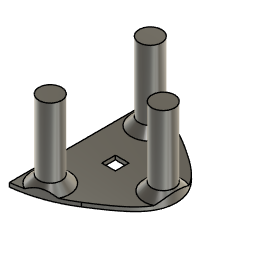
DirectionEncoderColumnSupport_PESTA (Autodesk Fusion 360 design; units mm, degrees)
Autodesk Fusion 360 part; units mm, degrees
note: some values were not read from the file. Set by a fixed rule: which sketch regions a step uses.
sketch "Sketch1" plane through (0, 0, 0) normal (0, 0, 1) x (1, 0, 0) in component "SuportePilarCentral"
  line L0 (39.35, 52.3) -> (-39.35, 52.3)
  line L1 (-39.35, 52.3) -> (-39.35, -52.3)
  line L2 (-39.35, -52.3) -> (39.35, -52.3)
  line L3 (39.35, -52.3) -> (39.35, 52.3)
  line L4 (39.35, 52.3) -> (-39.35, -52.3) construction
  line L5 (-39.35, 52.3) -> (39.35, -52.3) construction
  dimension "d1" = 78.7
  dimension "d2" = 104.6
  constraint horizontal L0
  constraint perpendicular L0 L1
  constraint parallel L0 L2
  constraint parallel L1 L3
  constraint coincident L4 origin
  constraint coincident L5 origin
  measures "d1" distance of L1.end L2.end
  measures "d2" distance of L0.end L1.end
extrude "Extrude1" add sketch "Sketch1" along normal blind 3 in component "SuportePilarCentral"
sketch "Sketch2" plane through (0, 0, 3) normal (0, 0, 1) x (-1, 0, 0) in component "SuportePilarCentral"
  line L0 (-39.35, 52.3) -> (-39.35, -52.3)
  line L1 (-39.35, -52.3) -> (39.35, -52.3)
  line L2 (39.35, -52.3) -> (39.35, 52.3)
  line L3 (39.35, 52.3) -> (-39.35, 52.3)
  circle A0 centre (23.55, -37.5) radius 8.5
  circle A1 centre (23.55, 37.5) radius 8.5
  line L4 (23.55, 37.5) -> (-23.65, 0)
  line L5 (-23.65, 0) -> (23.55, -37.5)
  circle A2 centre (-23.65, 0) radius 8.5
  dimension "d5" = 17
  dimension "d6" = 17
  dimension "d8" = 14.8
  dimension "d10" = 75
  dimension "d11" = 15.8
  dimension "d12" = 15.7
  dimension "d13" = 14.8
  dimension "d14" = 17
  constraint vertical A0.centre A1.centre
  constraint coincident A1.centre L4.start
  constraint coincident A0.centre L5.end
  constraint equal L4 L5
  constraint coincident L4.end L5.start
  measures "d5" diameter of A0
  measures "d6" diameter of A1
  measures "d8" distance of L3 A1.centre
  measures "d10" distance of A0.centre A1.centre
  measures "d11" distance of L2 A0.centre
  measures "d12" distance of L0 L4.end
  measures "d13" distance of L1 A0.centre
  measures "d14" diameter of A2
extrude "Extrude2" add sketch "Sketch2" along normal blind 58 contours A0 | A1 | L4 L5 A2 | L4 L5 A2 in component "SuportePilarCentral"
sketch "Sketch3" plane through (0, 0, 3) normal (0, 0, 1) x (-1, 0, 0) in component "SuportePilarCentral"
  circle A0 centre (23.55, 37.5) radius 8.5
  circle A1 centre (-23.65, 0) radius 8.5
  circle A2 centre (23.55, -37.5) radius 8.5
  line L0 (-39.35, 52.3) -> (-39.35, -52.3)
  line L1 (-39.35, -52.3) -> (39.35, -52.3)
  line L2 (39.35, -52.3) -> (39.35, 52.3)
  line L3 (39.35, 52.3) -> (-39.35, 52.3)
  spline S0 degree 5 poles (22.6923, -52.3) (20.9712, -51.282) (17.5667, -49.2595) (12.5727, -46.2662) (6.1404, -42.3567) (-1.5034, -37.5955) (-8.7027, -32.927) (-15.368, -28.2811) (-21.358, -23.5391) (-26.4613, -18.515) (-30.4038, -12.9641) (-32.9147, -6.7761) (-33.7822, 0) (-32.9147, 6.7761) (-30.4038, 12.9641) (-26.4613, 18.515) (-21.358, 23.5391) (-15.368, 28.2811) (-8.7027, 32.927) (-1.5034, 37.5955) (6.1404, 42.3567) (12.5727, 46.2662) (17.5667, 49.2595) (20.9712, 51.282) (22.6923, 52.3) knots 0 0 0 0 0 0 0.05 0.1 0.15 0.2 0.25 0.3 0.35 0.4 0.45 0.5 0.55 0.6 0.65 0.7 0.75 0.8 0.85 0.9 0.95 1 1 1 1 1 1
  line L4 (-33.35, -11.7865) -> (-33.35, 11.7865)
  point P0 (-19.35, -25)
  point P1 (-33.35, 0)
  point P2 (-19.35, 25)
  dimension "d17" = 25
  dimension "d18" = 25
  dimension "d19" = 6
  dimension "d20" = 20
  constraint coincident L1 S0.start
  constraint coincident L3 S0.end
  constraint vertical P0 P2
  constraint midpoint P1 L4
  constraint vertical L4
  constraint horizontal origin P1
  measures "d17" vertical distance of P0 P1
  measures "d18" vertical distance of P1 P2
  measures "d19" distance of L0 P1
  measures "d20" distance of L0 P0
extrude "Extrude3" cut sketch "Sketch3" against normal blind 3 contours L0 L1 L3 S0 in component "SuportePilarCentral"
fillet "Fillet1" radius 95 2 edges at (-22.6923, 52.3, 1.5) (-22.6923, -52.3, 1.5) in component "SuportePilarCentral"
sketch "Sketch4" plane through (0, 0, 3) normal (0, 0, 1) x (-1, 0, 0) in component "SuportePilarCentral"
  spline S0 degree 3 poles (-0.4688, 38.2043) (5.5357, 42.0059) (11.9479, 45.1218) (25.3467, 49.8648) (32.291, 51.4772) (39.35, 52.3) knots 0 0 0 0 2.132026 2.132026 4.264052 4.264052 4.264052 4.264052
  spline S1 degree 5 poles (-0.4688, 38.2043) (-0.6541, 38.087) (-2.3306, 37.0243) (-5.4453, 35.0269) (-9.8704, 32.1131) (-15.368, 28.2811) (-21.358, 23.5391) (-26.4613, 18.515) (-30.4038, 12.9641) (-32.9147, 6.7761) (-33.7822, 0) (-32.9147, -6.7761) (-30.4038, -12.9641) (-26.4613, -18.515) (-21.358, -23.5391) (-15.368, -28.2811) (-9.8704, -32.1131) (-5.4453, -35.0269) (-2.3306, -37.0243) (-0.6541, -38.087) (-0.4688, -38.2043) knots -0.856201 -0.856201 -0.856201 -0.856201 -0.856201 -0.856201 -0.85 -0.8 -0.75 -0.7 -0.65 -0.6 -0.55 -0.5 -0.45 -0.4 -0.35 -0.3 -0.25 -0.2 -0.15 -0.143799 -0.143799 -0.143799 -0.143799 -0.143799 -0.143799
  spline S2 degree 3 poles (39.35, -52.3) (37.5871, -52.0945) (34.0728, -51.5847) (28.8525, -50.5259) (23.6998, -49.1763) (18.6307, -47.5402) (13.6612, -45.6227) (8.8069, -43.4298) (4.0831, -40.9685) (1.0308, -39.1537) (-0.4688, -38.2043) knots 0 0 0 0 0.125 0.25 0.375 0.5 0.625 0.75 0.875 1 1 1 1
  line L0 (39.35, -52.3) -> (39.35, 52.3)
  circle A0 centre (23.55, -37.5) radius 8.5
  circle A1 centre (-23.65, 0) radius 8.5
  circle A2 centre (23.55, 37.5) radius 8.5
  line L1 (17.35, -5.1) -> (7.15, -5.1)
  line L2 (7.15, -5.1) -> (7.15, 5.1)
  line L3 (7.15, 5.1) -> (17.35, 5.1)
  line L4 (17.35, 5.1) -> (17.35, -5.1)
  point P0 (7.15, 0)
  dimension "d25" = 10.2
  dimension "d26" = 10.2
  dimension "d27" = 22
  constraint horizontal L1
  constraint vertical L2
  constraint horizontal L3
  constraint vertical L4
  constraint midpoint L2 P0
  constraint horizontal origin P0
  measures "d25" distance of L1.start L1.end
  measures "d26" distance of L1.start L3.end
  measures "d27" distance of L0 L4
extrude "Extrude4" cut sketch "Sketch4" against normal blind 3 contours L1 L2 L3 L4 in component "SuportePilarCentral"
chamfer "Chamfer1" distance 6 angle 45 3 edges at (-15.6252, 34.4263, 3) (-15.6252, -40.5737, 3) (31.5748, -3.0737, 3) in component "SuportePilarCentral"
component "SuportePilarCentral" placed x (1, 0, 0) y (0, 1, 0) z (0, 0, 1) at (0, 0, 0)
equation "d8 = ( 17 / 2 ) * 1 mm + 6.3 mm"
equation "d10 = 92 mm - 17 mm"
equation "d11 = ( 17 / 2 ) * 1 mm + 7.3 mm"
equation "d12 = ( 17 / 2 ) * 1 mm + 7.2 mm"
